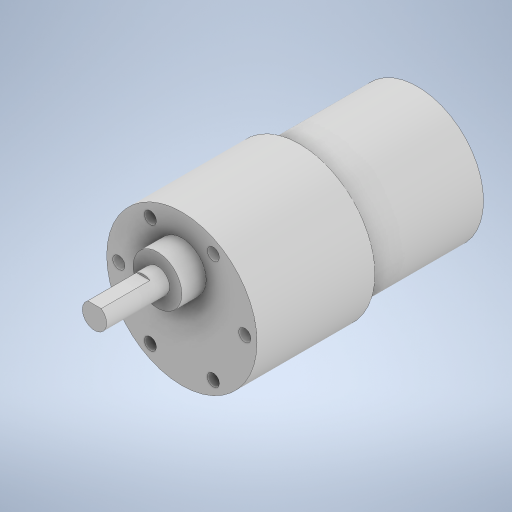
# Autodesk Inventor part: motor12kg
Saved by Autodesk Inventor 2024.3 (Build 283343000, 343)
## iProperties
Created: 2024-05-19
Part Number: motor12kg
Material: Generic
Document SubType Name: Modeling
Designer: USUARIO
Density: 1 g/cm^3
Appearance: Default
Author: USUARIO
Autodesk Inventor part; units mm, degrees
ref_plane "YZ Plane" through (0, 0, 0) normal (1, 0, 0) x (0, 1, 0)
ref_plane "XZ Plane" through (0, 0, 0) normal (0, 1, 0) x (-1, 0, 0)
ref_plane "XY Plane" through (0, 0, 0) normal (0, 0, 1) x (1, 0, 0)
sketch "Sketch1" plane through (0, 0, 0) normal (0, 0, 1) x (1, 0, 0)
  circle A0 centre (0, 0) radius 18.5
  line L0 (0, 0) -> (0, 7) construction
  circle A1 centre (0, 7) radius 6
  dimension "d0" = 37
  dimension "d1" = 7
  dimension "d2" = 12
  constraints: 2 centre point, 2 coincident, 2 end point, 1 vertical
  measures "d0" diameter of A0
  measures "d1" distance of L0.start L0.end
  measures "d2" diameter of A1
extrude "Extrusion1" add sketch "Sketch1" against normal blind 29 contours A0 | A1
extrude "Extrusion2" add sketch "Sketch1" along normal blind 6 contours A1
sketch "Sketch2" plane through (0, 7, 6) normal (0, 0, 1) x (1, 0, 0)
  circle A0 centre (0, 0) radius 3
  point P0 (0, -7)
  dimension "d7" = 6
  constraints: 1 centre point
  measures "d7" diameter of A0
extrude "Extrusion3" add sketch "Sketch2" along normal blind 15.5
sketch "Sketch3" plane through (0, 0, -29) normal (0, 0, -1) x (-1, 0, 0)
  circle A0 centre (0, 0) radius 16.25
  dimension "d10" = 32.5
  constraints: 1 centre point, 1 coincident
  measures "d10" diameter of A0
extrude "Extrusion4" add sketch "Sketch3" along normal blind 29
sketch "Sketch4" plane through (0, 7, 21.5) normal (0, 0, 1) x (1, 0, 0)
  circle A0 centre (0, 0) radius 3 projected
  arc A1 (-1.6583, 2.5) -> (1.6583, 2.5) centre (0, 0) ccw
  line L0 (-4.0487, 2.5) -> (4.6782, 2.5)
  arc A2 (1.6583, 2.5) -> (-1.6583, 2.5) centre (0, 0) ccw
  point P0 (0, -7)
  point P1 (0, -3)
  point P2 (-1.6583, 2.5)
  point P3 (1.6583, 2.5)
  dimension "d13" = 6
  dimension "d14" = 5.5
  constraints: 4 point on circle, 2 centre point, 2 end point, 2 point on line, 1 coincident, 1 horizontal, 2 other
  measures "d13" diameter of A1
  measures "d14" distance from line of L0 point (0, -3)
extrude "Extrusion5" cut sketch "Sketch4" against normal blind 12 contours L0 A0 picked at (-0.1169, 2.6598)
sketch "Sketch5" plane through (0, 0, 0) normal (0, 0, 1) x (1, 0, 0)
  circle A0 centre (0, 0) radius 15.5 construction
  line L0 (-7.75, -13.4234) -> (12.777, 22.1304) construction
  line L1 (0, 0) -> (25.5539, 0) construction
  line L2 (7.75, -13.4234) -> (-11.3824, 19.7148) construction
  line L3 (0, 0) -> (22.7647, 0) construction
  circle A1 centre (-15.5, 0) radius 1.5
  circle A2 centre (-7.75, 13.4234) radius 1.5
  circle A3 centre (7.75, 13.4234) radius 1.5
  circle A4 centre (15.5, 0) radius 1.5
  circle A5 centre (7.75, -13.4234) radius 1.5
  circle A6 centre (-7.75, -13.4234) radius 1.5
  dimension "d17" = 31
  dimension "d18" = 60
  dimension "d19" = 120
  dimension "d20" = 3
  dimension "d21" = 3
  dimension "d22" = 3
  dimension "d23" = 3
  dimension "d24" = 3
  dimension "d25" = 3
  constraints: 8 end point, 7 centre point, 6 point on circle, 4 point on line, 3 coincident, 2 horizontal
  measures "d17" diameter of A0
  measures "d18" angle of L1 L0
  measures "d19" angle of L3 L2
  measures "d20" diameter of A1
  measures "d21" diameter of A2
  measures "d22" diameter of A3
  measures "d23" diameter of A4
  measures "d24" diameter of A5
  measures "d25" diameter of A6
extrude "Extrusion6" cut sketch "Sketch5" against normal blind 10
body "Solid1"
